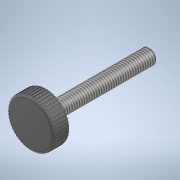
# Autodesk Inventor part: Thumbscrew - Long
Saved by Autodesk Inventor 2020 (Build 240168000, 168)
## iProperties
Created: 2020-02-14
Part Number: Thumbscrew - Long
Material: ABS Plastic
Document SubType Name: Modeling
Designer: Ishaan
Density: 1.06 g/cm^3
Appearance: Smooth - Black
Author: Ishaan
Autodesk Inventor part; units mm, degrees
ref_plane "YZ Plane" through (0, 0, 0) normal (1, 0, 0) x (0, 1, 0)
ref_plane "XZ Plane" through (0, 0, 0) normal (0, 1, 0) x (-1, 0, 0)
ref_plane "XY Plane" through (0, 0, 0) normal (0, 0, 1) x (1, 0, 0)
sketch "Sketch1" plane through (0, 0, 0) normal (0, 0, 1) x (1, 0, 0)
  circle A0 centre (0, 0) radius 4.8
  dimension "d0" = 9.6
  constraints: 1 centre point, 1 coincident
  measures "d0" diameter of A0
extrude "Extrusion1" add sketch "Sketch1" along normal blind 4.4
sketch "Sketch2" plane through (0, 0, 0) normal (0, 0, -1) x (-1, 0, 0)
  circle A0 centre (0, 0) radius 1.5
  dimension "d3" = 3
  constraints: 1 centre point, 1 coincident
  measures "d3" diameter of A0
extrude "Extrusion2" add sketch "Sketch2" along normal blind 20
sketch "Sketch3" plane through (0, 0, 0) normal (0, 0, -1) x (-1, 0, 0)
  circle A0 centre (0, 0) radius 1.5 projected
  circle A1 centre (0, 0) radius 4.8 projected
  circle A2 centre (0, 0) radius 3
  dimension "d7" = 6
  constraints: 1 centre point
  measures "d7" diameter of A2
extrude "Extrusion3" cut sketch "Sketch3" against normal blind 1 contours A1
chamfer "Chamfer1" distance 0.25 angle 45 1 edges at (1.5, 0, -20)
fillet "Fillet1" radius 0.5 2 edges at (-4.8, 0, 1) (-4.8, 0, 4.4)
fillet "Fillet2" radius 0.25 2 edges at (3, 0, 1) (3, 0, 0)
thread "Thread1" size "M3x0.5" class "6g" standard "ANSI Metric M Profile" full length
sketch "Sketch4" plane through (0, 0, 4.4) normal (0, 0, 1) x (1, 0, 0)
  circle A0 centre (0, 0) radius 4.3 projected
  circle A1 centre (0, 0) radius 4.3 projected
  circle A2 centre (0, 0) radius 4.3 projected
  circle A3 centre (0, 0) radius 4.3 projected
  circle A4 centre (0, 0) radius 4.8 projected
  line L0 (4.8, -0.125) -> (4.675, -0.125)
  line L1 (4.675, -0.125) -> (4.675, 0.125)
  line L2 (4.675, 0.125) -> (4.8, 0.125)
  line L3 (4.8, 0.125) -> (4.8, -0.125)
  line L4 (4.8, -0.125) -> (4.675, 0.125) construction
  line L5 (4.675, -0.125) -> (4.8, 0.125) construction
  point P0 (4.7375, 0)
  point P1 (4.7375, 0)
  dimension "d17" = 0.25
  dimension "d18" = 0.125
  constraints: 12 end point, 3 midpoint, 2 parallel, 1 horizontal, 1 horizontal alignment, 1 perpendicular, 1 tangent
  measures "d17" distance between parallel lines of L0 L2
  measures "d18" distance between parallel lines of L1 L3
extrude "Extrusion4" cut sketch "Sketch4" against normal through all contours A4 L0 L1 L2 picked at (4.7167, 0)
pattern_circular "Circular Pattern1" count 50 over 360 about axis through (0, 0, -10) along (0, 0, 1) of "Extrusion4"
body "Solid1"
